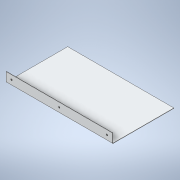
# Autodesk Inventor part: Separador
Saved by Autodesk Inventor 2021 (Build 250183000, 183)
## iProperties
Created: 2021-05-10
Part Number: Separador
Material: Steel ASTM A36
Document SubType Name: Sheet Metal
Designer: Nelson
Density: 7.85 g/cm^3
Sheet Metal Rule: Default_mm
Appearance: Plate
Flat Pattern Width: 22.3614 cm
Flat Pattern Length: 33.7 cm
Flat Pattern Area: 753.58 cm^2
Sheet Metal Width: 223,614 mm
Sheet Metal Length: 337,000 mm
Sheet Metal Area: 75358,031 mm^2
Mass: 709.677 g
Surface Area: 1520.77 cm^2
Volume: 90.4047 cm^3
Author: Nelson
Autodesk Inventor part; units mm, degrees
ref_plane "YZ Plane" through (0, 0, 0) normal (1, 0, 0) x (0, 1, 0)
ref_plane "XZ Plane" through (0, 0, 0) normal (0, 1, 0) x (-1, 0, 0)
ref_plane "XY Plane" through (0, 0, 0) normal (0, 0, 1) x (1, 0, 0)
sketch "Sketch2" plane through (0, 0, 0) normal (0, 1, 0) x (-1, 0, 0)
  line L0 (0, 0) -> (-337, 0)
  line L1 (-337, 0) -> (-337, -193)
  line L2 (-337, -193) -> (0, -193)
  line L3 (0, -193) -> (0, 0)
  dimension "d3" = 337
  dimension "d4" = 193
  measures "d3" distance of L0.start L0.end
  measures "d4" distance of L0.end L1.end
extrude "Plate1" add sketch "Sketch2" along normal blind 1.2
sketch "Sketch3" plane through (337, 2.4, 1.2) normal (0, 0, 1) x (1, 0, 0)
  line L0 (-337, 0) -> (0, 0)
  line L1 (0, 0) -> (0, 27.9)
  line L2 (0, 27.9) -> (-337, 27.9)
  line L3 (-337, 27.9) -> (-337, 0)
  constraints: 6 end point, 1 horizontal, 1 perpendicular, 1 vertical
edge flange "Flange1" height 30.3 angle 90 thickness 1.2 bend radius 1.2 thickness toward (0, 0, 1) relief straight relief width 1.2 relief depth 0.6 edges at (168.5, 1.2, 0) wall of the first edge with corners at (0, 2.4, 1.2) (337, 2.4, 1.2) (337, 30.3, 1.2) (0, 30.3, 1.2)
bend "Bend1"
corner "Corner1"
sketch "Sketch4" plane through (337, 30.3, 1.2) normal (0, 0, -1) x (-1, 0, 0)
  line L0 (337, 0) -> (337, -27.9) projected
  line L1 (0, 0) -> (0, -27.9) projected
  line L2 (337, 0) -> (0, 0) projected
  point P0 (337, -30.3)
  point P1 (320, -13.95)
  point P2 (168.5, -13.95)
  point P3 (17, -13.95)
  dimension "d16" = 17
  dimension "d17" = 17
  dimension "d18" = 151.5
  dimension "d19" = 13.95
  dimension "d20" = 13.95
  dimension "d21" = 13.95
  measures "d16" distance from line of point (320, -13.95) L0
  measures "d17" distance from line of L1 point (17, -13.95)
  measures "d18" distance of point (168.5, -13.95) point (320, -13.95)
  measures "d19" distance from line of L2 point (320, -13.95)
  measures "d20" distance from line of point (168.5, -13.95) L2
  measures "d21" distance from line of point (17, -13.95) L2
hole "Hole1" at (17, 16.35, 1.2) at (168.5, 16.35, 1.2) at (320, 16.35, 1.2) direction (0, 0, 1) diameter 5 depth 1.2 tip angle 118
equation "\"d17\" = d16"
equation "\"d20\" = d19"
equation "\"d21\" = d19"
equation "\"d27\" = Thickness"
equation "\"d5\" = Thickness"
equation "\"d6\" = BendReliefWidth"
equation "\"d7\" = BendReliefDepth"
equation "\"d8\" = MinimumRemnant"
equation "\"d9\" = TransitionRadius"
equation "\"d12\" = BendRadius"
equation "\"d13\" = CornerReliefSize"
equation "\"d14\" = GapSize"
equation "\"d15\" = JacobiRadiusSize"
equation "\"BendRadius\" = Thickness"
equation "\"BendReliefWidth\" = Thickness"
equation "\"BendReliefDepth\" = 0.5 * Thickness"
equation "\"CornerReliefSize\" = 4 * Thickness"
equation "\"MinimumRemnant\" = 2 * Thickness"
equation "\"TransitionRadius\" = BendRadius"
equation "\"JacobiRadiusSize\" = BendRadius"
equation "\"GapSize\" = Thickness"
equation "\"Thickness\" = 1.2"
body "Solid1"
